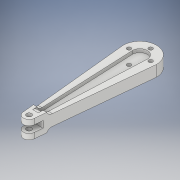
# Autodesk Inventor part: Delta_Arm
Saved by Autodesk Inventor 2019 (Build 230136000, 136)
## iProperties
Created: 2019-07-06
Part Number: Delta_Arm
Material: ABS Plastic
Document SubType Name: Modeling
Designer: Jorian Brusind
Density: 1.06 g/cm^3
Appearance: Smooth - White
Author: Jorian Brusind
Autodesk Inventor part; units mm, degrees
ref_plane "YZ Plane" through (0, 0, 0) normal (1, 0, 0) x (0, 1, 0)
ref_plane "XZ Plane" through (0, 0, 0) normal (0, 1, 0) x (-1, 0, 0)
sketch "Sketch1" plane through (0, 0, 0) normal (0, 1, 0) x (-1, 0, 0)
  circle A0 centre (0, 0) radius 5
  line L0 (0, 0) -> (0, -100)
  circle A1 centre (0, -100) radius 15
  line L1 (5, 0) -> (15, -100)
  line L2 (-5, 0) -> (-15, -100)
  dimension "d0" = 10
  dimension "d1" = 100
  dimension "d2" = 30
  dimension "d3" = 100
  dimension "d4" = 5.711
  dimension "d5" = 5.711
  dimension "d6" = 100
  constraints: 6 end point, 4 point on circle, 2 centre point, 2 coincident, 1 vertical
  measures "d0" diameter of A0
  measures "d1" distance of L0.start L0.end
  measures "d2" diameter of A1
  measures "d3" vertical distance of L1.start L1.end
  measures "d4" angle of L0 L1
  measures "d5" angle of L0 L2
  measures "d6" vertical distance of L2.start L2.end
extrude "Extrusion1" add sketch "Sketch1" along normal blind 10 contours A0 | L1 A1 L0 A0 | A0 L0 A1 L2 | L1 A1 L2
sketch "Sketch2" plane through (0, 10, 0) normal (0, 1, 0) x (1, 0, 0)
  circle A0 centre (0, 0) radius 2.25
  dimension "d9" = 4.5
  constraints: 1 centre point, 1 coincident
  measures "d9" diameter of A0
extrude "Extrusion2" cut sketch "Sketch2" against normal blind 10
sketch "Sketch3" plane through (0, 10, 0) normal (0, 1, 0) x (1, 0, 0)
  arc A0 (15, 100) -> (-15, 100) centre (0, 100) ccw projected
  circle A1 centre (0, 0) radius 2.25 projected
  line L0 (0, 0) -> (2.25, 0) construction
  line L1 (0, 100) -> (-6.75, 100)
  line L2 (0, 100) -> (6.75, 100) construction
  line L3 (0, 100) -> (6.75, 100)
  line L4 (6.75, 100) -> (2.25, 0)
  line L5 (-2.25, 0) -> (-6.75, 100)
  line L6 (0, 0) -> (-2.25, 0)
  line L7 (0, 0) -> (2.25, 0)
  arc A2 (6.75, 100) -> (-6.75, 100) centre (0, 100) ccw
  dimension "d15" = 2.25
  dimension "d16" = 6.75
  dimension "d17" = 180
  dimension "d18" = 2.25
  constraints: 16 end point, 4 horizontal, 3 collinear, 2 point on circle, 1 centre point, 1 coincident
  measures "d15" distance of L6.start L5.start
  measures "d16" distance of L1.start L1.end
  measures "d17" angle of L1 L2
  measures "d18" distance of L0.start L0.end
extrude "Extrusion3" cut sketch "Sketch3" against normal blind 3 contours L7 L6 A1 | A1 L5 L1 L3 L4 | L3 L1 A2 picked at (-1.4782, 0.1795)
sketch "Sketch4" plane through (0, 10, 0) normal (0, 1, 0) x (1, 0, 0)
  arc A0 (6.75, 100) -> (-6.75, 100) centre (0, 100) ccw projected
  line L0 (0, 100) -> (-9.779, 100)
  circle A1 centre (-9.779, 100) radius 1.75
  circle A2 centre (0, 109.779) radius 1.75
  circle A3 centre (9.779, 100) radius 1.75
  circle A4 centre (0, 90.221) radius 1.75
  point P0 (0, 0)
  dimension "d21" = 9.779
  dimension "d22" = 3.5
  dimension "d25" = 360
  constraints: 4 centre point, 2 end point, 1 coincident, 1 horizontal, 9 other
  measures "d21" distance of L0.start L0.end
  measures "d22" diameter of A1
extrude "Extrusion4" cut sketch "Sketch4" against normal blind 10
sketch "Sketch6" plane through (0, 0, 0) normal (0, -1, 0) x (1, 0, 0)
  arc A0 (-3.2257, -110.762) -> (3.2257, -110.762) centre (0, -109.779) ccw
  arc A1 (-9.0202, -104.6756) -> (-4.6756, -109.0202) centre (0, -100) ccw
  circle A2 centre (-9.779, 0) radius 1.5
  circle A3 centre (0, 9.779) radius 1.5
  arc A4 (-9.0202, -104.6756) -> (-10.762, -103.2257) centre (-11.6135, -106.0199) ccw
  arc A5 (-10.762, -96.7743) -> (-10.762, -103.2257) centre (-9.779, -100) ccw
  arc A6 (-3.2257, -110.762) -> (-4.6756, -109.0202) centre (-6.0199, -111.6135) ccw
  arc A7 (4.6756, -109.0202) -> (9.0202, -104.6756) centre (0, -100) ccw
  arc A8 (4.6756, -109.0202) -> (3.2257, -110.762) centre (6.0199, -111.6135) ccw
  arc A9 (10.762, -103.2257) -> (10.762, -96.7743) centre (9.779, -100) ccw
  arc A10 (10.762, -103.2257) -> (9.0202, -104.6756) centre (11.6135, -106.0199) ccw
  arc A11 (9.0202, -95.3244) -> (4.6756, -90.9798) centre (0, -100) ccw
  arc A12 (9.0202, -95.3244) -> (10.762, -96.7743) centre (11.6135, -93.9801) ccw
  arc A13 (3.2257, -89.238) -> (4.6756, -90.9798) centre (6.0199, -88.3865) ccw
  arc A14 (3.2257, -89.238) -> (-3.2257, -89.238) centre (0, -90.221) ccw
  arc A15 (-4.6756, -90.9798) -> (-9.0202, -95.3244) centre (0, -100) ccw
  arc A16 (-4.6756, -90.9798) -> (-3.2257, -89.238) centre (-6.0199, -88.3865) ccw
  arc A17 (-10.762, -96.7743) -> (-9.0202, -95.3244) centre (-11.6135, -93.9801) ccw
  circle A18 centre (0, -109.779) radius 1.75 projected
  dimension "d32" = 9.779
  constraints: 32 point on circle, 18 centre point
  measures "d32" distance of A18.centre A1.centre
extrude "Extrusion5" cut sketch "Sketch6" against normal blind 3 contours A6 A1 A4 A5 A17 A15 A16 A14 A13 A11 A12 A9 A10 A7 A8 A0
ref_plane "Work Plane1" through (0, 5, 0) normal (0, -1, 0) x (1, 0, 0)
mirror "Mirror1" about plane through (0, 5, 0) normal (0, -1, 0) of "Extrusion3"
sketch "Sketch7" plane through (0, 10, 0) normal (0, 1, 0) x (1, 0, 0)
  arc A0 (-2.25, 0) -> (2.25, 0) centre (0, 0) ccw projected
  circle A1 centre (0, 0) radius 2.25
  arc A2 (-5, 0) -> (5, 0) centre (0, 0) ccw projected
  circle A3 centre (0, 0) radius 5
  line L0 (-15, 100) -> (-5, 0) projected
  line L1 (-5, 0) -> (-5.995, 9.9504)
  line L2 (-6.3947, 92.1049) -> (-2.25, 0) projected
  line L3 (-2.4462, 4.3607) -> (-2.6978, 9.9504)
  line L4 (5, 0) -> (15, 100) projected
  line L5 (5, 0) -> (5.995, 9.9504)
  line L6 (6.3947, 92.1049) -> (2.25, 0) projected
  line L7 (2.4462, 4.3607) -> (2.6978, 9.9504)
  line L8 (5.995, 9.9504) -> (2.6978, 9.9504)
  line L9 (-2.6978, 9.9504) -> (-5.995, 9.9504)
  line L10 (-2.6978, 9.9504) -> (2.6978, 9.9504)
  dimension "d36" = 10
  dimension "d37" = 10
  constraints: 14 end point, 6 point on line, 3 point on circle, 2 coincident, 1 centre point, 1 collinear, 1 horizontal, 1 horizontal alignment, 2 other
  measures "d36" distance of L0.end L1.end
  measures "d37" distance of L4.start L5.end
extrude "Extrusion6" add sketch "Sketch7" along normal mid plane 6 contours L2 A3 L6 A1 | A0 L6 A3 A2 L2 | L2 L10 L6 A3 | A3 L0 L9 L2 | L6 L8 L4 A3
mirror "Mirror2" about plane through (0, 5, 0) normal (0, -1, 0) of "Extrusion6"
fillet "Fillet1" radius 5 3 edges at (0, 3, -9.9504) (4.3464, 0, -9.9504) (-4.3464, 0, -9.9504)
fillet "Fillet2" radius 5 3 edges at (-4.3464, 10, -9.9504) (4.3464, 10, -9.9504) (0, 7, -9.9504)
fillet "Fillet3" radius 5 2 edges at (0, 13, -9.9504) (0, -3, -9.9504)
ref_plane "Work Plane2" through (0, 0, 5) normal (0, 0, 1) x (1, 0, 0)
sketch "Sketch9" plane through (0, 0, 5) normal (0, 0, 1) x (1, 0, 0)
  line L0 (5, -3) -> (5, 13) projected
  line L1 (5, 5) -> (0, 5)
  line L2 (6, 8) -> (-6, 8)
  line L3 (-6, 8) -> (-6, 2)
  line L4 (-6, 2) -> (6, 2)
  line L5 (6, 2) -> (6, 8)
  line L6 (6, 8) -> (-6, 2) construction
  line L7 (-6, 8) -> (6, 2) construction
  point P0 (0, 0)
  dimension "d45" = 5
  dimension "d46" = 12
  dimension "d47" = 6
  constraints: 14 end point, 3 midpoint, 2 horizontal, 2 parallel, 1 perpendicular
  measures "d45" distance of L1.start L1.end
  measures "d46" distance of L4.end L3.end
  measures "d47" distance of L3.end L2.end
extrude "Extrusion7" cut sketch "Sketch9" against normal blind 12
body "Solid1"
